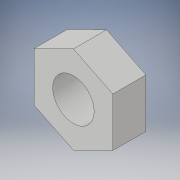
# Autodesk Inventor part: M5-nut
Saved by Autodesk Inventor 2018 (Build 220112000, 112)
## iProperties
Created: 2017-10-07
Part Number: M5-nut
Material: Generic
Document SubType Name: Modeling
Designer: Jurjen
Density: 1 g/cm^3
Appearance: Default
Author: Jurjen
Autodesk Inventor part; units mm, degrees
ref_plane "YZ Plane" through (0, 0, 0) normal (1, 0, 0) x (0, 1, 0)
ref_plane "XZ Plane" through (0, 0, 0) normal (0, 1, 0) x (-1, 0, 0)
ref_plane "XY Plane" through (0, 0, 0) normal (0, 0, 1) x (1, 0, 0)
sketch "Sketch1" plane through (0, 0, 0) normal (0, 0, 1) x (1, 0, 0)
  line L0 (-4.75, 2.9559) -> (0, 5.2945)
  line L1 (0, 5.2945) -> (4.75, 2.9559)
  line L2 (4.75, 2.9559) -> (4.75, -2.9559)
  line L3 (4.75, -2.9559) -> (0, -5.2945)
  line L4 (0, -5.2945) -> (-4.75, -2.9559)
  line L5 (-4.75, -2.9559) -> (-4.75, 2.9559)
  circle A0 centre (0, 0) radius 2.5
  circle A1 centre (0, 0) radius 4.75
  point P0 (4.75, 0)
  dimension "d6" = 5
  dimension "d8" = 9.5
  constraints: 12 end point, 3 horizontal alignment, 3 parallel, 2 centre point, 2 coincident, 2 tangent, 2 vertical alignment, 1 midpoint, 1 vertical
  measures "d6" diameter of A0
  measures "d8" diameter of A1
extrude "Extrusion1" add sketch "Sketch1" along normal blind 4
body "Solid1"
